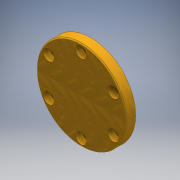
# Autodesk Inventor part: Крышка маленькая_62
Saved by Autodesk Inventor 2016 (Build 200138000, 138)
## iProperties
Created: 2021-04-23
Part Number: Крышка маленькая_62
Material: Типовые
Document SubType Name: Modeling
Designer: Лол
Density: 1 g/cm^3
Appearance: Сварка — латунь
Author: Лол
Autodesk Inventor part; units mm, degrees
ref_plane "YZ Plane" through (0, 0, 0) normal (1, 0, 0) x (0, 1, 0)
ref_plane "XZ Plane" through (0, 0, 0) normal (0, 1, 0) x (-1, 0, 0)
ref_plane "XY Plane" through (0, 0, 0) normal (0, 0, 1) x (1, 0, 0)
sketch "Эскиз1" plane through (0, 0, 0) normal (0, 0, 1) x (1, 0, 0)
  line L0 (0, 5) -> (0, 0)
  line L1 (0, 0) -> (31, 0)
  line L2 (31, 0) -> (31, 18)
  line L3 (31, 18) -> (26, 18)
  line L4 (26, 18) -> (26, 5)
  line L5 (26, 5) -> (0, 5)
  dimension "d0" = 18
  dimension "d1" = 5
  dimension "d3" = 31
  constraints: 12 end point, 5 perpendicular, 1 parallel, 1 vertical
  measures "d0" distance of L1.end L2.end
  measures "d1" distance of L2.end L3.end
  measures "d3" distance of L0.end L1.end
revolve "Вращение1" add sketch "Эскиз1" angle 360 about axis through (0, 5, 0) along (0, -1, 0)
sketch "Эскиз2" plane through (0, 0, 0) normal (1, 0, 0) x (0, 1, 0)
  line L0 (0, 31) -> (0, -31) projected
  line L1 (18, 31) -> (0, 31) projected
  line L2 (18, 31) -> (0, 31) projected
  line L3 (0, 0) -> (0, 45)
  line L4 (0, 45) -> (10, 45)
  line L5 (10, 45) -> (10, 0)
  line L6 (10, 0) -> (0, 0)
  line L7 (-4.2, 0) -> (25.2, 0) projected
  dimension "d5" = 10
  dimension "d6" = 45
  constraints: 8 end point, 2 perpendicular, 1 point on line, 1 vertical
  measures "d5" distance of L3.end L4.end
  measures "d6" distance between parallel lines of L6 L4
revolve "Вращение2" add sketch "Эскиз2" angle 360 about axis through (0, -10, 0) along (0, 1, 0)
sketch "Эскиз3" plane through (0, 0, 0) normal (0, -1, 0) x (1, 0, 0)
  line L0 (0, -63) -> (0, 63) projected
  line L1 (-63, 0) -> (63, 0) projected
  circle A0 centre (0, 0) radius 37.5 construction
  circle A1 centre (0, 37.5) radius 5.5
  dimension "d8" = 75
  dimension "d9" = 11
  constraints: 2 coincident, 1 centre point, 1 point on line, 1 vertical alignment, 2 other
  measures "d9" diameter of A1
hole "Отверстие1" at (0, 0, 37.5) direction (0, 1, 0) diameter 6.2 depth 15 tip angle 118 counterbore diameter 11 counterbore depth 6.8
pattern_circular "Круговой массив1" count 6 over 360 about axis through (0, -10, 0) along (0, 1, 0) of "Отверстие1"
fillet "Сопряжение1" radius 1.3 1 edges at (-31, 10, 0)
chamfer "Фаска1" distance 1 angle 45 1 edges at (0, 0, -45)
chamfer "Фаска2" distance 2 angle 45 1 edges at (-31, 18, 0)
